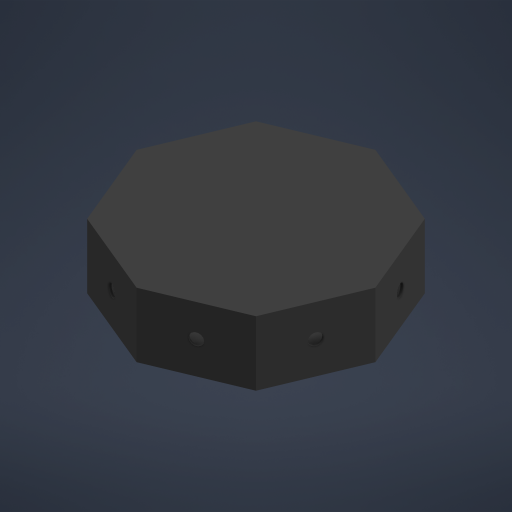
# Autodesk Inventor part: board_case
Saved by Autodesk Inventor 2023 (Build 270158000, 158)
## iProperties
Created: 2022-05-01
Part Number: board_case
Material: PVC, Unplasticized
Document SubType Name: Modeling
Designer: Norbert Ligas
Density: 1.29 g/cm^3
Appearance: Rubber - Black
diameter: 200,000 mm
bar_diameter: 8,000 mm
outher_heigth: 54,000 mm
inner_heigth: 50,000 mm
thickness: 2,000 mm
inner_diameter: 196,000 mm
Author: Norbert Ligas
Autodesk Inventor part; units mm, degrees
note: some values were not read from the file. Chosen so that the rebuilt part matches the saved one: direction of "Hole1".
ref_plane "YZ Plane" through (0, 0, 0) normal (1, 0, 0) x (0, 1, 0)
ref_plane "XY Plane" through (0, 0, 0) normal (0, 0, 1) x (1, 0, 0)
sketch "Sketch1" plane through (0, 0, 0) normal (0, 1, 0) x (1, 0, 0)
  line L0 (70.7107, 70.7107) -> (-70.7107, -70.7107) construction
  line L1 (-70.7107, 70.7107) -> (70.7107, -70.7107) construction
  line L2 (-140, 0) -> (140, 0) construction
  line L3 (0, -140) -> (0, 140) construction
  line L4 (100, 0) -> (70.7107, 70.7107)
  line L5 (0, 100) -> (70.7107, 70.7107)
  line L6 (-70.7107, 70.7107) -> (0, 100)
  line L7 (-70.7107, 70.7107) -> (-100, 0)
  line L8 (-100, 0) -> (-70.7107, -70.7107)
  line L9 (-70.7107, -70.7107) -> (0, -100)
  line L10 (0, -100) -> (70.7107, -70.7107)
  line L11 (70.7107, -70.7107) -> (100, 0)
  line L12 (0, 100) -> (0, -100) construction
  line L13 (-100, 0) -> (100, 0) construction
  line L14 (98, 0) -> (69.2965, 69.2965)
  line L15 (0, 98) -> (69.2965, 69.2965)
  line L16 (0, 98) -> (-69.2965, 69.2965)
  line L17 (-69.2965, 69.2965) -> (-98, 0)
  line L18 (-98, 0) -> (-69.2965, -69.2965)
  line L19 (-69.2965, -69.2965) -> (0, -98)
  line L20 (0, -98) -> (69.2965, -69.2965)
  line L21 (69.2965, -69.2965) -> (98, 0)
  point P0 (0, 0)
  point P1 (0, 0)
  dimension "d0" = 45
  dimension "d3" = 200
  dimension "d6" = 2
  constraints: 44 end point, 12 point on line, 7 parallel, 6 midpoint, 3 equal length, 3 perpendicular, 1 symmetric about line
  measures "d0" angle of L2 L0
  measures "d3" distance of L4.start L7.end
  measures "d6" distance of L4.start L14.start
extrude "Extrusion1" add sketch "Sketch1" along normal blind 54
extrude "Extrusion2" add sketch "Sketch1" along normal blind 2 contours L11 L10 L9 L8 L7 L6 L5 L4 | L21 L20 L19 L18 L17 L16 L15 L14
ref_plane "Work Plane4" through (-100, 54, 0) normal (0, 1, 0) x (-1, 0, 0)
sketch "Sketch3" plane through (-100, 54, 0) normal (0, 1, 0) x (-1, 0, 0)
  line L0 (-29.2893, -70.7107) -> (0, 0) projected
  line L1 (-100, -100) -> (-29.2893, -70.7107) projected
  line L2 (-170.7107, -70.7107) -> (-100, -100) projected
  line L3 (-200, 0) -> (-170.7107, -70.7107) projected
  line L4 (-170.7107, 70.7107) -> (-200, 0) projected
  line L5 (-100, 100) -> (-170.7107, 70.7107) projected
  line L6 (-29.2893, 70.7107) -> (-100, 100) projected
  line L7 (0, 0) -> (-29.2893, 70.7107) projected
  point P0 (-100, 0)
extrude "Extrusion4" add sketch "Sketch3" against normal blind 2
sketch "Sketch4" plane through (0, 0, 100) normal (0.3826834, 0, 0.9238795) x (0.9238795, 0, -0.3826834)
  line L0 (76.5367, 54) -> (0, 54) projected
  line L1 (38.2683, 54) -> (38.2683, 0) construction
  line L2 (76.5367, 0) -> (0, 0) projected
  line L3 (75.7713, 2) -> (0.7654, 2) construction
  point P0 (38.2683, 27)
  dimension "d15" = 25
  constraints: 2 end point, 2 midpoint, 1 perpendicular
  measures "d15" distance from line of L3 point (38.268, 27)
hole "Hole1" at (35.3553, 27, 85.3553) direction (-0.3826834, 0, -0.9238795) diameter 10 depth 1.8478
pattern_circular "Circular Pattern1" count 8 over 360 about axis through (0, -10, 0) along (0, 1, 0) of "Hole1"
equation "\"d3\" = diameter"
equation "\"d6\" = thickness"
equation "\"d7\" = outher_heigth"
equation "\"d9\" = thickness"
equation "\"d13\" = thickness"
equation "\"d15\" = hole_pos_y"
equation "\"d16\" = hole_diameter"
equation "\"diameter\" = 200"
equation "\"inner_diameter\" = diameter - 2 * thickness"
equation "\"thickness\" = 2"
equation "\"inner_heigth\" = 50"
equation "\"outher_heigth\" = inner_heigth + 2 * thickness"
equation "\"hole_pos_y\" = 0.5 * inner_heigth"
equation "\"hole_diameter\" = 10"
body "Solid1"
